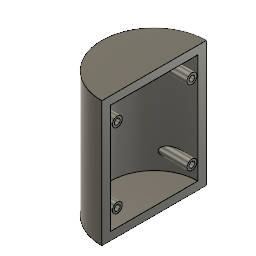
Robot Shell v1 (Autodesk Fusion 360 design; units mm, degrees)
Autodesk Fusion 360 part; units mm, degrees
sketch "Sketch1" plane through (0, 0, 0) normal (0, 1, 0) x (1, 0, 0)
  circle A0 centre (0, 0) radius 31.75
  dimension "d1" = 63.5
  constraint coincident A0.centre origin
  measures "d1" diameter of A0
extrude "Extrude1" add sketch "Sketch1" along normal blind 76.2
sketch "Sketch2" plane through (0, 76.2, 0) normal (0, 1, 0) x (-1, 0, 0)
  circle A0 centre (0, 0) radius 31.75
  circle A1 centre (0, 0) radius 27.94
  dimension "d4" = 55.88
  constraint concentric A0 A1
  measures "d4" diameter of A1
extrude "Extrude2" cut sketch "Sketch2" against normal blind 80 contours A1
sketch "Sketch3" plane through (0, 76.2, 0) normal (0, 1, 0) x (-1, 0, 0)
  circle A0 centre (0, 0) radius 27.94
  circle A1 centre (0, 0) radius 31.75
  line L0 (0, 0) -> (0, -31.75)
  line L1 (0, 0) -> (0, 31.75)
  line L2 (0, 31.75) -> (0, -31.75)
  line L3 (0, 31.75) -> (0, -31.75)
  constraint coincident A0.centre A1.centre
  constraint coincident A1 L0.end
  constraint vertical L0
  constraint coincident A1 L1.end
  constraint parallel L0 L1
  constraint parallel L2 L3
extrude "Extrude3" cut sketch "Sketch3" against normal blind 80 contours A0 A1 L0 L1 L2 L3 picked at (-19.495, -23.3296)
sketch "Sketch4" plane through (0, 0, 0) normal (1, 0, 0) x (0, 0, -1)
  circle A0 centre (22.859, 60.5719) radius 3
  circle A1 centre (22.859, 15.3599) radius 3
  circle A2 centre (-22.353, 60.5719) radius 3
  circle A3 centre (-22.353, 15.3599) radius 3
  circle A4 centre (22.859, 60.5719) radius 1.75
  circle A5 centre (22.859, 15.3599) radius 1.75
  circle A6 centre (-22.353, 15.3599) radius 1.75
  circle A7 centre (-22.353, 60.5719) radius 1.75
  dimension "d23" = 6
  dimension "d24" = 6
  dimension "d25" = 6
  dimension "d26" = 6
  dimension "d27" = 3.5
  dimension "d28" = 3.5
  dimension "d29" = 3.5
  dimension "d30" = 3.5
  constraint concentric A0 A4
  constraint concentric A1 A5
  constraint concentric A3 A6
  constraint concentric A2 A7
  measures "d23" diameter of A0
  measures "d24" diameter of A1
  measures "d25" diameter of A2
  measures "d26" diameter of A3
  measures "d27" diameter of A4
  measures "d28" diameter of A5
  measures "d29" diameter of A6
  measures "d30" diameter of A7
extrude "Extrude4" add sketch "Sketch4" against normal blind 18
sketch "Sketch5" plane through (0, 76.2, 0) normal (0, 1, 0) x (-1, 0, 0)
  line L0 (0, -27.94) -> (0, -31.75)
  arc A0 (0, -31.75) -> (0, 31.75) centre (0, 0) ccw
  line L1 (0, 31.75) -> (0, 27.94)
  arc A1 (0, -27.94) -> (0, 27.94) centre (0, 0) ccw
  circle A2 centre (0, 0) radius 29.845
  circle A3 centre (0, 0) radius 26.449
  line L2 (0, -29.845) -> (0, 29.845)
  constraint concentric A0 A2
  constraint concentric A0 A3
  constraint midpoint L0 L2.start
  constraint midpoint L1 L2.end
extrude "Extrude5" add sketch "Sketch5" against normal blind 76.2 contours A1 A3 L2
sketch "Sketch6" plane through (0, 76.2, 0) normal (0, 1, 0) x (-1, 0, 0)
  line L0 (0, -26.449) -> (0, -31.75)
  arc A0 (0, -31.75) -> (0, 31.75) centre (0, 0) ccw
  line L1 (0, 31.75) -> (0, 26.449)
  arc A1 (0, -26.449) -> (0, 26.449) centre (0, 0) ccw
  circle A2 centre (0, 0) radius 26.449
  line L2 (0, -26.449) -> (0, 26.449)
  constraint concentric A0 A2
  constraint coincident L0.start A2
  constraint coincident L0.start A1.start
  constraint coincident L1.end A1.end
extrude "Extrude6" add sketch "Sketch6" against normal blind 5 contours A1 A2 L2
sketch "Sketch7" plane through (0, 0, 0) normal (0, -1, 0) x (1, 0, 0)
  line L0 (0, -31.75) -> (0, -26.449)
  arc A0 (0, 26.449) -> (0, -26.449) centre (0, 0) ccw
  line L1 (0, 26.449) -> (0, 31.75)
  arc A1 (0, 31.75) -> (0, -31.75) centre (0, 0) ccw
  line L2 (0, -26.449) -> (0, 26.449)
  circle A2 centre (0, 0) radius 26.449
  line L3 (0, 26.449) -> (0, -26.449)
  constraint coincident L0.end A0.end
  constraint coincident A0.start L1.start
  constraint coincident A0.centre A1.centre
  constraint coincident A0.start A2
  constraint parallel L2 L3
extrude "Extrude7" add sketch "Sketch7" against normal blind 5 contours A0 L2 A2 L3
